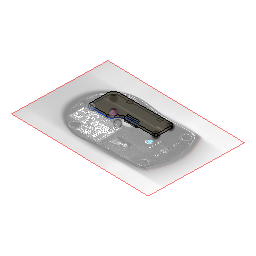
P1 - Tapa ratón a partir de escaneo terminada (Autodesk Fusion 360 design; units mm, degrees)
Autodesk Fusion 360 part; units mm, degrees
sketch "Sketch1" plane through (0, 0, 0) normal (0, 0, 1) x (1, 0, 0)
  line L0 (0, 0) -> (35.2, 0)
  line L1 (36.7, 1.5) -> (36.7, 14)
  line L2 (35.2, 15.5) -> (-10.6, 15.5)
  line L3 (-15.6, 10.5) -> (-15.6, -4.583)
  line L4 (-14.1, -6.083) -> (0, -6.083)
  line L5 (0, -6.083) -> (0, 0)
  arc A0 (9.8843, 0) -> (4.2448, -3.4707) centre (9.8843, -6.3171) ccw
  arc A1 (0, -6.083) -> (4.2448, -3.4707) centre (0, -1.3282) ccw
  arc A2 (-15.6, -4.583) -> (-14.1, -6.083) centre (-14.1, -4.583) ccw
  arc A3 (36.7, 14) -> (35.2, 15.5) centre (35.2, 14) ccw
  arc A4 (35.2, 0) -> (36.7, 1.5) centre (35.2, 1.5) ccw
  arc A5 (-10.6, 15.5) -> (-15.6, 10.5) centre (-10.6, 10.5) ccw
  line L6 (26.7, 15.5) -> (26.7, 17)
  line L7 (26.7, 17) -> (23.7, 17)
  line L8 (23.7, 17) -> (23.7, 15.5)
  line L9 (-2.6, 15.5) -> (-2.6, 17)
  line L10 (-2.6, 17) -> (0.4, 17)
  line L11 (0.4, 17) -> (0.4, 15.5)
  line L12 (9.4567, -0.0145) -> (9.4567, -0.5)
  line L13 (9.4567, -0.5) -> (19.7509, -0.5)
  line L14 (19.7509, -0.5) -> (19.7509, 0)
  line L15 (-2.6, 15.5) -> (-2.6, 13.5)
  line L16 (-2.6, 13.5) -> (0.4, 13.5)
  line L17 (0.4, 13.5) -> (0.4, 15.5)
  line L18 (23.7, 15.5) -> (23.7, 13.5)
  line L19 (23.7, 13.5) -> (26.7, 13.5)
  line L20 (26.7, 13.5) -> (26.7, 15.5)
  line L21 (9.4567, -0.0145) -> (9.4567, 2.9855)
  line L22 (9.4567, 2.9855) -> (19.7509, 2.9855)
  line L23 (19.7509, 2.9855) -> (19.7509, 0)
  line L24 (9.4567, 1.4855) -> (19.7509, 1.4928)
  dimension "d1" = 1.5
  dimension "d2" = 5
  dimension "d3" = 52.3
  dimension "d4" = 1.5
  dimension "d5" = 3
  dimension "d6" = 10
  dimension "d7" = 1.5
  dimension "d8" = 3
  dimension "d9" = 13
  dimension "d10" = 15.5
  dimension "d11" = 15.6
  dimension "d12" = 0.5
  dimension "d13" = 2
  dimension "d14" = 2
  dimension "d15" = 3
  constraint coincident L0.start L5.end
  constraint horizontal L0
  constraint perpendicular L0 L1
  constraint perpendicular L1 L2
  constraint perpendicular L2 L3
  constraint perpendicular L3 L4
  constraint perpendicular L0 L5
  constraint tangent L0 A0
  constraint coincident L0 A0.start
  constraint tangent L4 A1
  constraint tangent A0 A1
  constraint tangent L3 A2
  constraint tangent L4 A2
  constraint tangent L2 A3
  constraint tangent L1 A3
  constraint equal A2 A3
  constraint tangent L1 A4
  constraint tangent L0 A4
  constraint equal A2 A4
  constraint tangent L2 A5
  constraint tangent L3 A5
  constraint coincident L2 L6.start
  constraint perpendicular L2 L6
  constraint perpendicular L6 L7
  constraint coincident L2 L8.end
  constraint perpendicular L2 L8
  constraint coincident L2 L9.start
  constraint perpendicular L2 L9
  constraint perpendicular L9 L10
  constraint coincident L2 L11.end
  constraint perpendicular L2 L11
  constraint coincident A0 L12.start
  constraint perpendicular L0 L12
  constraint perpendicular L12 L13
  constraint coincident L0 L14.end
  constraint perpendicular L0 L14
  constraint parallel L9 L15
  constraint perpendicular L11 L16
  constraint perpendicular L2 L17
  constraint perpendicular L2 L18
  constraint perpendicular L6 L19
  constraint perpendicular L19 L20
  constraint perpendicular L0 L21
  constraint perpendicular L14 L22
  constraint perpendicular L0 L23
  constraint midpoint L21 L24.start
  constraint midpoint L23 L24.end
  measures "d1" radius of A2
  measures "d2" radius of A5
  measures "d3" distance of L1 L3
  measures "d4" distance of L6.start L6.end
  measures "d5" distance of L6.end L7.end
  measures "d6" distance of L1 L6
  measures "d7" distance of L10.end L11.end
  measures "d8" distance of L9.end L10.end
  measures "d9" distance of L3 L9
  measures "d10" distance of L0 L2
  measures "d11" distance of L0.start L3
  measures "d12" distance of L13.end L14.end
  measures "d13" distance of L11.end L16.end
  measures "d14" distance of L8.end L18.end
  measures "d15" distance of L12.start L21.end
extrude "Extrude1" add sketch "Sketch1" along normal blind 2 contours L0 L21 L23 L24 | L0 L1 L2 L3 L4 L5 A2 A3 A4 A5 L15 L16 L17 L18 L19 L20 L21 L22 L23 | L0 L5 A0 A1 L21 | L2 L18 L19 L20 | L2 L15 L16 L17 makes body 1
extrude "Extrude2" add sketch "Sketch1" against normal blind 1.5 separate body contours L0 L21 L23 L24 | L0 A0 L12 L13 L14 | L2 L18 L19 L20 | L2 L6 L7 L8 | L2 L15 L16 L17 | L2 L9 L10 L11 makes body 2 at (-0.6, 15.8333, 0) makes body 3 at (16.462, 0.3309, 0) makes body 4 at (24.7, 15.8333, 0)
combine "Combine1" operation add target body 1 tool bodies 3 2 4
chamfer "Chamfer1" distance 0.5 angle 45 6 edges at (25.2, 17, -1.5) (-1.1, 17, -1.5) (14.6038, -0.5, -1.5) (-1.1, 13.5, -1.5) (25.2, 13.5, -1.5) (14.6038, 1.4891, -1.5) on bodies 1
fillet "Fillet1" radius 0.5 6 edges at (-2.6, 17, -0.5) (0.4, 17, -0.5) (23.7, 17, -0.5) (26.7, 17, -0.5) (19.7509, -0.5, -0.5) (9.4567, -0.5, -0.5) on bodies 1
named bodies: "tapa ratón"
